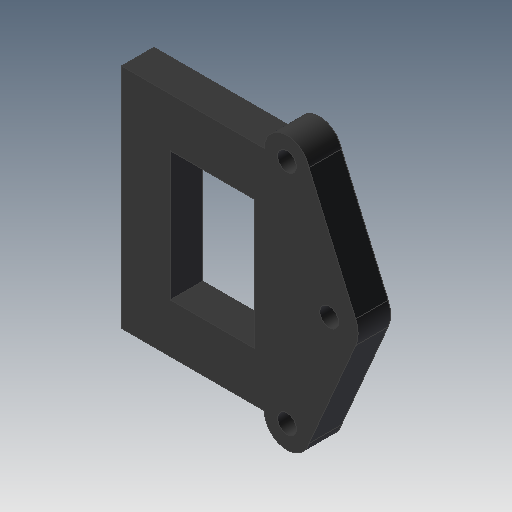
# Autodesk Inventor part: 03_OTmic_belt_gear
Saved by Autodesk Inventor 2019.4 (Build 234330000, 330)
## iProperties
Created: 2020-10-07
Part Number: 03_OTmic_belt_gear
Material: Generic
Document SubType Name: Modeling
Designer: diederichbenedict
Density: 1 g/cm^3
Appearance: Default
Author: diederichbenedict
Autodesk Inventor part; units mm, degrees
ref_plane "YZ Plane" through (0, 0, 0) normal (1, 0, 0) x (0, 1, 0)
ref_plane "XZ Plane" through (0, 0, 0) normal (0, 1, 0) x (-1, 0, 0)
ref_plane "XY Plane" through (0, 0, 0) normal (0, 0, 1) x (1, 0, 0)
sketch "Sketch1" plane through (0, 0, 0) normal (0, 0, 1) x (1, 0, 0)
  circle A0 centre (11.5096, -17.4937) radius 1.45 projected
  circle A1 centre (11.4904, 17.5063) radius 1.45 projected
  line L0 (-6.5054, 9.9465) -> (-6.4946, -9.9535) projected
  line L1 (-6.4946, -9.9535) -> (6.5054, -9.9465) projected
  line L2 (6.5054, -9.9465) -> (6.4946, 9.9535) projected
  line L3 (6.4946, 9.9535) -> (-6.5054, 9.9465) projected
  arc A2 (8.0096, -17.4956) -> (11.0077, -14.0299) centre (11.5096, -17.4937) ccw projected
  line L4 (8.0096, -17.4956) -> (-13.9904, -17.5076) projected
  line L5 (-13.9904, -17.5076) -> (-14.0096, 17.4924) projected
  line L6 (-14.0096, 17.4924) -> (7.9904, 17.5044) projected
  arc A3 (10.9923, 14.0419) -> (7.9904, 17.5044) centre (11.4904, 17.5063) ccw projected
  line L7 (10.9923, 14.0419) -> (11.0077, -14.0299) projected
  ellipse E0 centre (120.0743, 0.0597) end of major axis (125.4052, -3.3899) minor radius 6.3497 projected
  circle A4 centre (18, 0.0098) radius 1.45
  line L8 (7.9904, 17.5044) -> (8.0096, -17.4956)
  circle A5 centre (18, 0.0098) radius 4.45
  line L9 (14.8825, 18.3689) -> (22.0821, 1.7816)
  line L10 (14.8825, -18.4283) -> (22.0851, -1.7549)
  point P0 (0, 0)
  dimension "d0" = 2.9
  dimension "d1" = 3
  dimension "d2" = 7
  constraints: 6 end point, 4 point on circle, 2 centre point, 2 tangent, 1 other
  measures "d0" diameter of A4
  measures "d1" radial gap between concentric circles of A4 A5
  measures "d2" distance from line of A4.centre L7
extrude "Extrusion1" add sketch "Sketch1" along normal blind 5 contours L8 A3 L7 A2 | L4 L5 L6 L8 | A2 L7 A3 L9 A5 L10 | A5
body "Solid1"
